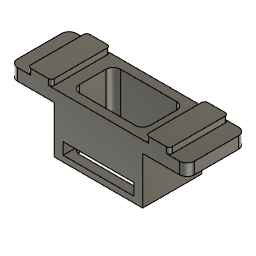
HP-001 (Autodesk Fusion 360 design; units mm, degrees)
Autodesk Fusion 360 part; units mm, degrees
sketch "Sketch1" plane through (0, 0, 0) normal (0, 0, 1) x (1, 0, 0) in component "Headpost"
  line L0 (7.5, -5) -> (-7.5, -5)
  line L1 (-7.5, -5) -> (-7.5, 5)
  line L2 (-7.5, 5) -> (7.5, 5)
  line L3 (7.5, 5) -> (7.5, -5)
  line L4 (7.5, -5) -> (-7.5, 5) construction
  line L5 (-7.5, -5) -> (7.5, 5) construction
  dimension "d1" = 15
  dimension "d2" = 10
  constraint horizontal L0
  constraint perpendicular L0 L1
  constraint parallel L0 L2
  constraint parallel L1 L3
  constraint coincident L4 origin
  constraint coincident L5 origin
  measures "d1" distance of L1.end L2.end
  measures "d2" distance of L0.end L1.end
extrude "Extrude1" add sketch "Sketch1" along normal blind 10 in component "Headpost"
sketch "Sketch2" plane through (0, 0, 10) normal (0, 0, 1) x (-1, 0, 0) in component "Headpost"
  line L0 (-7.5, -5) -> (7.5, -5)
  line L1 (7.5, -5) -> (7.5, 5)
  line L2 (7.5, 5) -> (-7.5, 5)
  line L3 (-7.5, 5) -> (-7.5, -5)
  line L4 (6, 3.5) -> (-6, 3.5)
  line L5 (-6, 3.5) -> (-6, -3.5)
  line L6 (-6, -3.5) -> (6, -3.5)
  line L7 (6, -3.5) -> (6, 3.5)
  dimension "d5" = -1.5
extrude "Extrude2" cut sketch "Sketch2" against normal blind 15 contours L4 L5 L6 L7 in component "Headpost"
sketch "Sketch3" plane through (-7.5, 0, 0) normal (-1, 0, 0) x (0, -1, 0) in component "Headpost"
  line L0 (-5, 0) -> (5, 0)
  line L1 (5, 0) -> (5, 10)
  line L2 (5, 10) -> (-5, 10)
  line L3 (-5, 10) -> (-5, 0)
  line L4 (-5, 10) -> (5, 10)
  line L5 (5, 10) -> (5, 8)
  line L6 (5, 8) -> (-5, 8)
  line L7 (-5, 8) -> (-5, 10)
  dimension "d8" = 10
  dimension "d9" = 2
  constraint horizontal L4
  constraint vertical L5
  constraint horizontal L6
  constraint vertical L7
  constraint coincident L2.end L3.start
  measures "d8" distance of L2.end L1.end
  measures "d9" distance of L2.end L6.end
extrude "Extrude3" add sketch "Sketch3" along normal blind 7.5 contours L1 L2 L3 L4 L5 L6 L7 in component "Headpost"
sketch "Sketch4" plane through (7.5, 0, 0) normal (1, 0, 0) x (0, 1, 0) in component "Headpost"
  line L0 (-5, 0) -> (5, 0)
  line L1 (5, 0) -> (5, 10)
  line L2 (5, 10) -> (-5, 10)
  line L3 (-5, 10) -> (-5, 0)
  line L4 (-5, 10) -> (5, 10)
  line L5 (5, 10) -> (5, 8)
  line L6 (5, 8) -> (-5, 8)
  line L7 (-5, 8) -> (-5, 10)
  dimension "d12" = 2
  constraint horizontal L4
  constraint vertical L5
  constraint horizontal L6
  constraint vertical L7
  constraint coincident L2.end L3.start
  measures "d12" distance of L2.end L6.end
extrude "Extrude4" add sketch "Sketch4" along normal blind 7.5 contours L1 L2 L3 L4 L5 L6 L7 in component "Headpost"
fillet "Fillet1" radius 1.25 2 edges at (6, -3.5, 5) (6, 3.5, 5) in component "Headpost"
fillet "Fillet2" radius 1.25 2 edges at (-6, 3.5, 5) (-6, -3.5, 5) in component "Headpost"
fillet "Fillet3" radius 1.25 4 edges at (15, -5, 9) (15, 5, 9) (-15, 5, 9) (-15, -5, 9) in component "Headpost"
sketch "Sketch5" plane through (0, 0, 10) normal (0, 0, 1) x (-1, 0, 0) in component "Headpost"
  arc A0 (15, 3.75) -> (13.75, 5) centre (13.75, 3.75) ccw
  line L0 (13.75, 5) -> (-13.75, 5)
  arc A1 (-13.75, 5) -> (-15, 3.75) centre (-13.75, 3.75) ccw
  line L1 (-15, 3.75) -> (-15, -3.75)
  arc A2 (-15, -3.75) -> (-13.75, -5) centre (-13.75, -3.75) ccw
  line L2 (-13.75, -5) -> (13.75, -5)
  arc A3 (13.75, -5) -> (15, -3.75) centre (13.75, -3.75) ccw
  line L3 (15, -3.75) -> (15, 3.75)
  line L4 (-4.75, 3.5) -> (4.75, 3.5)
  arc A4 (6, 2.25) -> (4.75, 3.5) centre (4.75, 2.25) ccw
  line L5 (6, 2.25) -> (6, -2.25)
  arc A5 (4.75, -3.5) -> (6, -2.25) centre (4.75, -2.25) ccw
  line L6 (4.75, -3.5) -> (-4.75, -3.5)
  arc A6 (-6, -2.25) -> (-4.75, -3.5) centre (-4.75, -2.25) ccw
  line L7 (-6, -2.25) -> (-6, 2.25)
  arc A7 (-4.75, 3.5) -> (-6, 2.25) centre (-4.75, 2.25) ccw
  line L8 (12, -5) -> (8, -5)
  line L9 (8, -5) -> (8, 5)
  line L10 (8, 5) -> (12, 5)
  line L11 (12, 5) -> (12, -5)
  line L12 (-8, -5) -> (-12, -5)
  line L13 (-12, -5) -> (-12, 5)
  line L14 (-12, 5) -> (-8, 5)
  line L15 (-8, 5) -> (-8, -5)
  dimension "d21" = 4
  dimension "d22" = 10
  dimension "d23" = 2
  dimension "d24" = 4
  dimension "d25" = 10
  dimension "d26" = 2
  constraint horizontal L8
  constraint vertical L9
  constraint horizontal L10
  constraint vertical L11
  constraint coincident L2 L8.start
  constraint horizontal L12
  constraint vertical L13
  constraint horizontal L14
  constraint vertical L15
  constraint coincident L2 L12.start
  measures "d21" distance of L8.start L8.end
  measures "d22" distance of L8.start L10.end
  measures "d23" distance of L5 L9
  measures "d24" distance of L12.start L12.end
  measures "d25" distance of L12.start L14.end
  measures "d26" distance of L7 L15
extrude "Extrude5" add sketch "Sketch5" along normal blind 1 contours L0 L2 L8 L9 L10 L11 in component "Headpost"
sketch "Sketch6" plane through (0, 0, 10) normal (0, 0, 1) x (-1, 0, 0) in component "Headpost"
  line L0 (-4.75, 3.5) -> (4.75, 3.5)
  arc A0 (6, 2.25) -> (4.75, 3.5) centre (4.75, 2.25) ccw
  line L1 (6, 2.25) -> (6, -2.25)
  arc A1 (4.75, -3.5) -> (6, -2.25) centre (4.75, -2.25) ccw
  line L2 (4.75, -3.5) -> (-4.75, -3.5)
  arc A2 (-6, -2.25) -> (-4.75, -3.5) centre (-4.75, -2.25) ccw
  line L3 (-6, -2.25) -> (-6, 2.25)
  arc A3 (-4.75, 3.5) -> (-6, 2.25) centre (-4.75, 2.25) ccw
  line L4 (8, -5) -> (8, 5)
  line L5 (8, 5) -> (-13.75, 5)
  arc A4 (-13.75, 5) -> (-15, 3.75) centre (-13.75, 3.75) ccw
  line L6 (-15, 3.75) -> (-15, -3.75)
  arc A5 (-15, -3.75) -> (-13.75, -5) centre (-13.75, -3.75) ccw
  line L7 (-13.75, -5) -> (8, -5)
  line L8 (-8, -5) -> (-12, -5)
  line L9 (-12, -5) -> (-12, 5)
  line L10 (-12, 5) -> (-8, 5)
  line L11 (-8, 5) -> (-8, -5)
  dimension "d29" = 4
  dimension "d30" = 10
  dimension "d31" = 2
  constraint horizontal L8
  constraint vertical L9
  constraint horizontal L10
  constraint vertical L11
  constraint coincident L7 L8.start
  measures "d29" distance of L8.start L8.end
  measures "d30" distance of L8.start L10.end
  measures "d31" distance of L3 L11
extrude "Extrude6" add sketch "Sketch6" along normal blind 1 contours L5 L7 L8 L9 L10 L11 in component "Headpost"
fillet "Fillet4" radius 0.5 2 edges at (-12, -5, 10.5) (-8, -5, 10.5) in component "Headpost"
fillet "Fillet5" radius 0.5 2 edges at (8, -5, 10.5) (12, -5, 10.5) in component "Headpost"
fillet "Fillet6" radius 0.5 2 edges at (12, 5, 10.5) (8, 5, 10.5) in component "Headpost"
fillet "Fillet7" radius 0.5 2 edges at (-8, 5, 10.5) (-12, 5, 10.5) in component "Headpost"
sketch "Sketch7" plane through (0, 5, 0) normal (0, 1, 0) x (-1, 0, 0) in component "Headpost"
  line L0 (13.75, 10) -> (11.5, 10)
  line L1 (11.5, 10) -> (11.5, 11)
  line L2 (11.5, 11) -> (8.5, 11)
  line L3 (8.5, 11) -> (8.5, 10)
  line L4 (8.5, 10) -> (-8.5, 10)
  line L5 (-8.5, 10) -> (-8.5, 11)
  line L6 (-8.5, 11) -> (-11.5, 11)
  line L7 (-11.5, 11) -> (-11.5, 10)
  line L8 (-11.5, 10) -> (-13.75, 10)
  line L9 (-13.75, 10) -> (-13.75, 8)
  line L10 (-13.75, 8) -> (-7.5, 8)
  line L11 (-7.5, 8) -> (-7.5, 0)
  line L12 (-7.5, 0) -> (7.5, 0)
  line L13 (7.5, 0) -> (7.5, 8)
  line L14 (7.5, 8) -> (13.75, 8)
  line L15 (13.75, 8) -> (13.75, 10)
  line L16 (-6, 3) -> (6, 3)
  line L17 (6, 3) -> (6, 1)
  line L18 (6, 1) -> (-6, 1)
  line L19 (-6, 1) -> (-6, 3)
  dimension "d42" = 2
  constraint horizontal L16
  constraint vertical L17
  constraint horizontal L18
  constraint vertical L19
  measures "d42" distance of L16.start L18.end
extrude "Extrude7" cut sketch "Sketch7" against normal blind 3 contours L16 L17 L18 L19 in component "Headpost"
sketch "Sketch8" plane through (0, -5, 0) normal (0, -1, 0) x (1, 0, 0) in component "Headpost"
  line L0 (13.75, 10) -> (11.5, 10)
  line L1 (11.5, 10) -> (11.5, 11)
  line L2 (11.5, 11) -> (8.5, 11)
  line L3 (8.5, 11) -> (8.5, 10)
  line L4 (8.5, 10) -> (-8.5, 10)
  line L5 (-8.5, 10) -> (-8.5, 11)
  line L6 (-8.5, 11) -> (-11.5, 11)
  line L7 (-11.5, 11) -> (-11.5, 10)
  line L8 (-11.5, 10) -> (-13.75, 10)
  line L9 (-13.75, 10) -> (-13.75, 8)
  line L10 (-13.75, 8) -> (-7.5, 8)
  line L11 (-7.5, 8) -> (-7.5, 0)
  line L12 (-7.5, 0) -> (7.5, 0)
  line L13 (7.5, 0) -> (7.5, 8)
  line L14 (7.5, 8) -> (13.75, 8)
  line L15 (13.75, 8) -> (13.75, 10)
  line L16 (-6, 3) -> (6, 3)
  line L17 (6, 3) -> (6, 1)
  line L18 (6, 1) -> (-6, 1)
  line L19 (-6, 1) -> (-6, 3)
  dimension "d45" = 2
  constraint horizontal L16
  constraint vertical L17
  constraint horizontal L18
  constraint vertical L19
  measures "d45" distance of L16.start L18.end
extrude "Extrude8" cut sketch "Sketch8" against normal blind 3 contours L16 L17 L18 L19 in component "Headpost"
component "Headpost" placed x (1, 0, 0) y (0, 1, 0) z (0, 0, 1) at (0, 0, 0)
